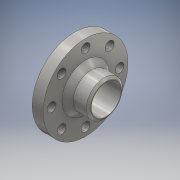
# Autodesk Inventor part: Flange 3 in
Saved by Autodesk Inventor 2016 (Build 200138000, 138)
## iProperties
Created: 2018-11-07
Part Number: Flange 3 in
Material: ASTM A105 Gr.B
Document SubType Name: Modeling
Designer: Wijaya
Mass: 6871.06 g
Surface Area: 1180.04 cm^2
Volume: 875.295 cm^3
Density: 7.85 g/cm^3
Appearance: Semi-Polished
Author: Wijaya
Autodesk Inventor part; units mm, degrees
note: some values were not read from the file. Chosen so that the rebuilt part matches the saved one: direction of "Hole1".
ref_plane "YZ Plane" through (0, 0, 0) normal (1, 0, 0) x (0, 1, 0)
ref_plane "XZ Plane" through (0, 0, 0) normal (0, 1, 0) x (-1, 0, 0)
ref_plane "XY Plane" through (0, 0, 0) normal (0, 0, 1) x (1, 0, 0)
sketch "Sketch1" plane through (0, 0, 0) normal (0, 0, 1) x (1, 0, 0)
  line L0 (0, 0) -> (109.4884, 0)
  line L1 (0, 36.83) -> (0, 58.5)
  line L2 (0, 58.5) -> (2, 58.5)
  line L3 (2, 58.5) -> (2, 105)
  line L4 (2, 105) -> (29, 105)
  line L5 (29, 105) -> (29, 58.5)
  line L6 (29, 58.5) -> (43.05, 44.45)
  line L7 (43.05, 44.45) -> (75.3807, 44.45)
  line L8 (75.3807, 44.45) -> (80, 38.43)
  line L9 (80, 38.43) -> (80, 36.83)
  line L10 (80, 36.83) -> (0, 36.83)
  point P0 (0, 47.665)
  dimension "d5" = 2
  dimension "d6" = 210
  dimension "d7" = 27
  dimension "d8" = 117
  dimension "d9" = 45
  dimension "d10" = 78
  dimension "d28" = 73.66
  dimension "d29" = 88.9
  dimension "d30" = 37.5
  dimension "d31" = 1.6
  constraints: 22 end point, 5 perpendicular, 1 horizontal, 1 midpoint, 1 parallel, 1 point on line, 1 vertical, 1 vertical alignment
  measures "d5" distance of L1.end L2.end
  measures "d6" diameter of L4 L0
  measures "d7" distance of L3.end L4.end
  measures "d8" diameter of L5.end L0
  measures "d9" angle of L7 L6
  measures "d10" distance from line of L3 L8.end
  measures "d28" diameter of L10 L0
  measures "d29" diameter of L7 L0
  measures "d30" angle of L9 L8
  measures "d31" distance of L8.end L9.end
revolve "Revolution1" add sketch "Sketch1" angle 360 about axis through (0, 0, 0) along (1, 0, 0)
sketch "Sketch2" plane through (2, 0, 0) normal (-1, 0, 0) x (0, 0, 1)
  point P0 (0, 0)
  point P1 (0, 84.14)
  dimension "d12" = 84.14
  constraints: 1 vertical alignment
  measures "d12" distance of point (0, 0) point (0, 84.14)
hole "Hole1" at (2, 84.14, 0) direction (1, 0, 0) diameter 22.225 end up to surface
pattern_circular "Circular Pattern1" count 8 over 360 about axis through (15.5, 0, 0) along (1, 0, 0) of "Hole1"
body "Solid1"
